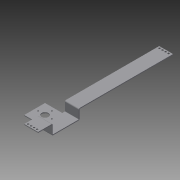
# Autodesk Inventor part: Cim Mount
Saved by Autodesk Inventor 2013 (Build 170138000, 138)
## iProperties
Created: 2013-01-24
Part Number: Cim Mount
Material: Generic
Document SubType Name: Sheet Metal
Designer: actoennies
Density: 1 g/cm^3
Sheet Metal Rule: Default
Mass: 102.418 g
Surface Area: 697.739 cm^2
Volume: 102.418 cm^3
Author: actoennies
Autodesk Inventor part; units mm, degrees
ref_plane "YZ Plane" through (0, 0, 0) normal (1, 0, 0) x (0, 1, 0)
ref_plane "XZ Plane" through (0, 0, 0) normal (0, 1, 0) x (-1, 0, 0)
ref_plane "XY Plane" through (0, 0, 0) normal (0, 0, 1) x (1, 0, 0)
sketch "Sketch1" plane through (0, 0, 0) normal (0, 1, 0) x (-1, 0, 0)
  circle A0 centre (0, -101.6) radius 2.5527
  circle A1 centre (25.4, -76.2) radius 2.5527
  circle A2 centre (50.8, -101.6) radius 2.5527
  circle A3 centre (25.4, -127) radius 2.5527
  line L0 (0, -139.7) -> (63.5, -139.7)
  line L1 (63.5, -139.7) -> (63.5, -63.5)
  line L2 (63.5, -63.5) -> (0, -63.5)
  circle A4 centre (25.4, -101.6) radius 12.7
  line L3 (0, -63.5) -> (0, -50.8)
  line L4 (0, -50.8) -> (-50.8, -50.8)
  line L5 (-50.8, -50.8) -> (-50.8, -152.4)
  line L6 (-50.8, -152.4) -> (0, -152.4)
  line L7 (0, -152.4) -> (0, -139.7)
  dimension "d0" = 25.4
  dimension "d1" = 25.4
  dimension "d2" = 25.4
  dimension "d3" = 12.7
  dimension "d4" = 50.8
  dimension "d5" = 50.8
  dimension "d6" = 12.7
  dimension "d7" = 50.8
  measures "d0" diameter of A4
  measures "d1" distance of A4.centre A0.centre
  measures "d2" distance of A3.centre A4.centre
  measures "d3" distance of L2.end L3.end
  measures "d4" distance of L3.end L4.end
  measures "d5" distance of L5.end L6.end
  measures "d6" distance of L6.end L0.start
  measures "d7" distance from line of A0.centre L5
extrude "Plate1" add sketch "Sketch1" along normal blind 3.175
sketch "Sketch2" plane through (50.8, 0, -53.975) normal (0, 0, 1) x (1, 0, 0)
  line L0 (-50.8, 0) -> (0, 0)
  line L1 (0, 0) -> (0, 38.1)
  line L2 (0, 38.1) -> (-50.8, 38.1)
  line L3 (-50.8, 38.1) -> (-50.8, 0)
  constraints: 6 end point, 1 horizontal, 1 perpendicular, 1 vertical
edge flange "Flange1" height 38.1 angle 90 thickness 3.175 bend radius 1.27 thickness toward (0, 0, 1) relief straight relief width 3.175 relief depth 1.5875 corner gap 3.175 corner form 0 edges at (25.4, 3.175, -50.8) (25.4, 3.175, -152.4) wall of the first edge with corners at (0, 0, -53.975) (50.8, 0, -53.975) (50.8, 38.1, -53.975) (0, 38.1, -53.975)
bend "Bend1"
corner "Corner1"
sketch "Sketch3" plane through (0, 38.1, -49.53) normal (0, -1, 0) x (1, 0, 0)
  line L0 (50.8, -1.27) -> (0, -1.27)
  line L1 (0, -1.27) -> (0, 49.53)
  line L2 (0, 49.53) -> (50.8, 49.53)
  line L3 (50.8, 49.53) -> (50.8, -1.27)
  constraints: 8 end point
edge flange "Flange2" height 53.975 angle 90 thickness 3.175 bend radius 1.27 thickness toward (0, -1, 0) relief straight relief width 3.175 relief depth 1.5875 edges at (25.4, 38.1, -50.8) wall of the first edge with corners at (50.8, 38.1, -50.8) (0, 38.1, -50.8) (0, 38.1, 0) (50.8, 38.1, 0)
bend "Bend2"
corner "Corner2"
sketch "Sketch4" plane through (50.8, 38.1, -153.67) normal (0, -1, 0) x (1, 0, 0)
  line L0 (-50.8, 1.27) -> (0, 1.27)
  line L1 (0, 1.27) -> (0, -341.63)
  line L2 (0, -341.63) -> (-50.8, -341.63)
  line L3 (-50.8, -341.63) -> (-50.8, 1.27)
  constraints: 8 end point
edge flange "Flange3" height 346.075 angle 90 thickness 3.175 bend radius 1.27 thickness toward (0, -1, 0) relief straight relief width 3.175 relief depth 1.5875 edges at (25.4, 38.1, -152.4) wall of the first edge with corners at (0, 38.1, -152.4) (50.8, 38.1, -152.4) (50.8, 38.1, -495.3) (0, 38.1, -495.3)
bend "Bend3"
corner "Corner3"
sketch "Sketch5" plane through (0, 38.1, 0) normal (0, 1, 0) x (1, 0, 0)
  line L0 (0, 153.67) -> (50.8, 153.67) projected
  line L1 (50.8, 495.3) -> (50.8, 153.67) projected
  line L2 (0, 495.3) -> (50.8, 495.3) projected
  line L3 (0, 153.67) -> (0, 495.3) projected
  circle A0 centre (7.8014, 488.95) radius 3.3782 projected
  circle A1 centre (18.8686, 488.95) radius 3.3782 projected
  circle A2 centre (29.9357, 488.95) radius 3.3782 projected
  circle A3 centre (41.0029, 488.95) radius 3.3782 projected
  circle A4 centre (7.8014, 6.35) radius 3.3782 projected
  circle A5 centre (18.8686, 6.35) radius 3.3782 projected
  circle A6 centre (29.9357, 6.35) radius 3.3782 projected
  circle A7 centre (41.0029, 6.35) radius 3.3782 projected
extrude "Cut1" cut sketch "Sketch5" against normal blind 3.175 contours A0 | A1 | A2 | A3 | A4 | A5 | A6 | A7
equation "\"d39\" = Thickness"
equation "\"d9\" = BendReliefWidth"
equation "\"d10\" = BendReliefDepth"
equation "\"d11\" = MinimumRemnant"
equation "\"d12\" = BendRadius"
equation "\"d16\" = CornerReliefSize"
equation "\"d17\" = GapSize"
equation "\"d18\" = JacobiRadiusSize"
equation "\"d19\" = BendReliefWidth"
equation "\"d20\" = BendReliefDepth"
equation "\"d21\" = MinimumRemnant"
equation "\"d22\" = BendRadius"
equation "\"d26\" = CornerReliefSize"
equation "\"d27\" = GapSize"
equation "\"d28\" = JacobiRadiusSize"
equation "\"d29\" = BendReliefWidth"
equation "\"d30\" = BendReliefDepth"
equation "\"d31\" = MinimumRemnant"
equation "\"d32\" = BendRadius"
equation "\"d36\" = CornerReliefSize"
equation "\"d37\" = GapSize"
equation "\"d38\" = JacobiRadiusSize"
equation "\"BendRadius\" = Thickness"
equation "\"BendReliefWidth\" = Thickness"
equation "\"BendReliefDepth\" = 0.5 * Thickness"
equation "\"CornerReliefSize\" = 4 * Thickness"
equation "\"MinimumRemnant\" = 2 * Thickness"
equation "\"TransitionRadius\" = BendRadius"
equation "\"JacobiRadiusSize\" = BendRadius"
equation "\"GapSize\" = Thickness"
equation "\"d8\" = BendRadius"
equation "\"Thickness\" = 3.175"
body "Solid1"
